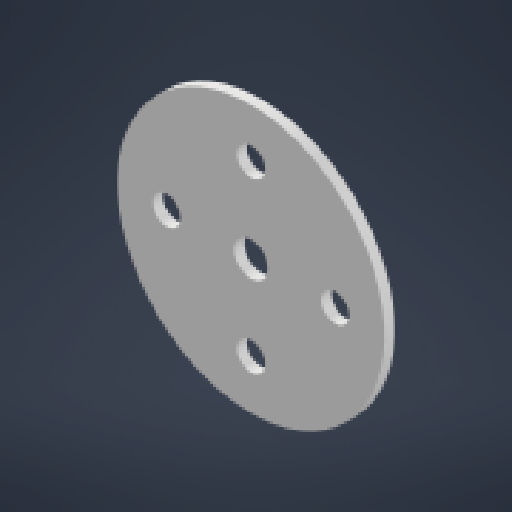
# Autodesk Inventor part: HS adapter retainer
Saved by Autodesk Inventor 2023.2 (Build 272271000, 271)
## iProperties
Created: 2023-03-21
Part Number: HS adapter retainer
Material: Generic
Document SubType Name: Modeling
Designer: Liam
Density: 1 g/cm^3
Appearance: Default
Author: Liam
Autodesk Inventor part; units mm, degrees
ref_plane "YZ Plane" through (0, 0, 0) normal (1, 0, 0) x (0, 1, 0)
ref_plane "XZ Plane" through (0, 0, 0) normal (0, 1, 0) x (-1, 0, 0)
ref_plane "XY Plane" through (0, 0, 0) normal (0, 0, 1) x (1, 0, 0)
sketch "Sketch1" plane through (0, 0, 0) normal (0, 0, 1) x (1, 0, 0)
  circle A0 centre (0, 12.7) radius 2.1
  circle A1 centre (12.7, 0) radius 2.1
  circle A2 centre (0, -12.7) radius 2.1
  circle A3 centre (-12.7, 0) radius 2.1
  circle A4 centre (0, 0) radius 2.54
  arc A5 (5.5881, 19.3163) -> (4.8187, 19.5224) centre (0, 0) ccw projected
  circle A6 centre (0, 0) radius 20.1083
  point P0 (5.5881, 19.3163)
  dimension "d0" = 5.08
  constraints: 5 centre point, 2 coincident, 7 other
  measures "d0" diameter of A4
extrude "Extrusion1" add sketch "Sketch1" along normal blind 1.524
body "Solid1"
